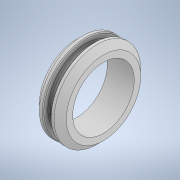
# Autodesk Inventor part: 72. Муфта синхронизатора
Saved by Autodesk Inventor 2021 (Build 250183000, 183)
## iProperties
Created: 2021-03-24
Part Number: 72. Муфта синхронизатора
Material: Типовые
Document SubType Name: Modeling
Designer: Данил
Density: 1 g/cm^3
Appearance: По умолчанию
Author: Данил
Autodesk Inventor part; units mm, degrees
ref_plane "YZ Plane" through (0, 0, 0) normal (1, 0, 0) x (0, 1, 0)
ref_plane "XZ Plane" through (0, 0, 0) normal (0, 1, 0) x (-1, 0, 0)
ref_plane "XY Plane" through (0, 0, 0) normal (0, 0, 1) x (1, 0, 0)
sketch "Эскиз1" plane through (0, 0, 0) normal (0, 0, 1) x (1, 0, 0)
  line L0 (-16.5, 0) -> (16.5, 0)
  line L1 (-16.5, -37.7) -> (-16.5, -45.5)
  line L2 (-16.5, -45.5) -> (-9, -53)
  line L3 (-9, -53) -> (-5.5, -53)
  line L4 (-16.5, -37.7) -> (16.5, -37.7)
  line L5 (16.5, -37.7) -> (16.5, -45.5)
  line L6 (16.5, -45.5) -> (9, -53)
  line L7 (9, -53) -> (5.5, -53)
  line L8 (4.5, -52) -> (4.5, -47.1)
  line L9 (2.9, -45.5) -> (-2.9, -45.5)
  line L10 (-4.5, -47.1) -> (-4.5, -52)
  arc A0 (-2.9, -45.5) -> (-4.5, -47.1) centre (-2.9, -47.1) ccw
  arc A1 (4.5, -47.1) -> (2.9, -45.5) centre (2.9, -47.1) ccw
  line L11 (5.5, -53) -> (4.5, -52)
  line L12 (-5.5, -53) -> (-4.5, -52)
  point P0 (0, 0)
  point P1 (0, 0)
  point P2 (-4.5, -53)
  point P3 (4.5, -53)
  point P4 (4.5, -45.5)
  point P5 (-4.5, -45.5)
  point P6 (0, -45.5)
  dimension "d0" = 33
  dimension "d1" = 106
  dimension "d2" = 91
  dimension "d3" = 45
  dimension "d4" = 75.4
  dimension "d5" = 9
  dimension "d6" = 1.6
  dimension "d9" = 45
  dimension "d10" = 1
  dimension "d11" = 45
  dimension "d12" = 1
  dimension "d13" = 45
  constraints: 26 end point, 8 point on line, 4 horizontal alignment, 4 perpendicular, 4 point on circle, 4 tangent, 3 vertical, 3 vertical alignment, 2 centre point, 2 horizontal, 2 midpoint, 1 coincident, 1 equal radius
  measures "d0" distance of L0.start L0.end
  measures "d1" diameter of L3 L0
  measures "d2" diameter of L1.end L0
  measures "d3" angle of L3 L2
  measures "d4" diameter of L1.start L0
  measures "d5" distance of point (4.5, -45.5) point (-4.5, -45.5)
  measures "d6" radius of A0
  measures "d9" angle of L7 L6
  measures "d10" distance of L7.end point (4.5, -53)
  measures "d11" angle of L7 L11
  measures "d12" distance of L3.end point (-4.5, -53)
  measures "d13" angle of L3 L12
revolve "Вращение1" add sketch "Эскиз1" angle 360 about axis through (-16.5, 0, 0) along (1, 0, 0)
equation "\"d12\" = d10"
equation "\"d13\" = d11"
